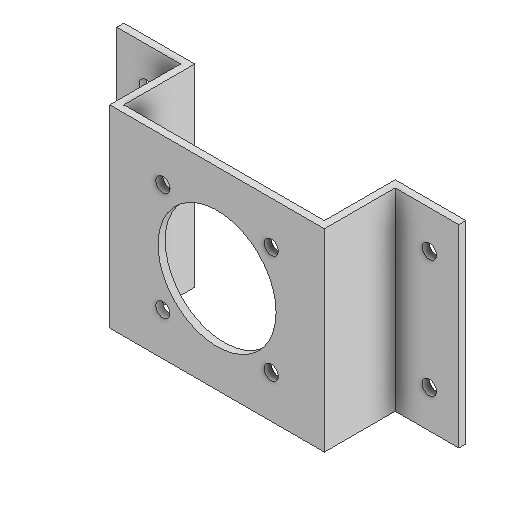
# Autodesk Inventor part: TopMotorBracket
Saved by Autodesk Inventor 2022 (Build 260153000, 153)
## iProperties
Created: 2024-07-02
Part Number: TopMotorBracket
Material: Generic
Document SubType Name: Modeling
Designer: LaptopJR
Density: 1 g/cm^3
Appearance: Default
Author: LaptopJR
Autodesk Inventor part; units mm, degrees
ref_plane "YZ Plane" through (0, 0, 0) normal (1, 0, 0) x (0, 1, 0)
ref_plane "XZ Plane" through (0, 0, 0) normal (0, 1, 0) x (-1, 0, 0)
ref_plane "XY Plane" through (0, 0, 0) normal (0, 0, 1) x (1, 0, 0)
sketch "Sketch1" plane through (0, 0, 0) normal (0, 1, 0) x (-1, 0, 0)
  line L0 (0, 0) -> (-30, 0)
  line L1 (-30, 0) -> (-30, 30)
  line L2 (-30, 30) -> (-115, 30)
  line L3 (-115, 30) -> (-115, 0)
  line L4 (-115, 0) -> (-145, 0)
  line L5 (0, 3) -> (-27, 3)
  line L6 (-27, 3) -> (-27, 33)
  line L7 (-27, 33) -> (-118, 33)
  line L8 (-118, 33) -> (-118, 3)
  line L9 (-118, 3) -> (-145, 3)
  line L10 (0, 0) -> (0, 3)
  line L11 (-145, 0) -> (-145, 3)
  dimension "d0" = 30
  dimension "d1" = 30
  dimension "d2" = 3
  dimension "d28" = 85
  constraints: 24 end point, 6 perpendicular, 2 point on line, 2 vertical, 1 collinear, 1 horizontal, 4 other
  measures "d0" distance of L0.start L0.end
  measures "d1" distance of L0.end L1.end
  measures "d2" distance between parallel lines of L2 L7
  measures "d28" distance of L1.end L2.end
extrude "Extrusion1" add sketch "Sketch1" along normal blind 82
sketch "Sketch2" plane through (27, 0, 33) normal (0, 0, 1) x (1, 0, 0)
  line L0 (0, 82) -> (91, 82) projected
  line L1 (45.5, 82) -> (45.5, 0) construction
  line L2 (0, 0) -> (91, 0) projected
  circle A0 centre (45.5, 41) radius 32.5 construction
  line L3 (45.5, 41) -> (68.481, 63.981) construction
  circle A1 centre (68.481, 63.981) radius 3.05
  circle A2 centre (22.519, 63.981) radius 3.05
  circle A3 centre (22.519, 18.019) radius 3.05
  circle A4 centre (68.481, 18.019) radius 3.05
  circle A5 centre (45.5, 41) radius 25.0125
  point P0 (-27, 0)
  dimension "d6" = 65
  dimension "d7" = 6.1
  dimension "d8" = 45
  dimension "d11" = 360
  dimension "d15" = 50.025
  constraints: 5 centre point, 4 end point, 3 midpoint, 2 coincident, 12 other
  measures "d7" diameter of A1
  measures "d8" angle of L1 L3
  measures "d15" diameter of A5
extrude "Extrusion2" cut sketch "Sketch2" against normal blind 82
sketch "Sketch3" plane through (0, 0, 3) normal (0, 0, 1) x (1, 0, 0)
  circle A0 centre (72.5, 41) radius 25.0125 construction
  line L0 (12.5, 66) -> (132.5, 66) construction
  line L1 (132.5, 66) -> (132.5, 16) construction
  line L2 (132.5, 16) -> (12.5, 16) construction
  line L3 (12.5, 16) -> (12.5, 66) construction
  line L4 (12.5, 66) -> (132.5, 16) construction
  line L5 (132.5, 66) -> (12.5, 16) construction
  circle A1 centre (12.5, 66) radius 3.05
  circle A2 centre (12.5, 16) radius 3.05
  circle A3 centre (132.5, 66) radius 3.05
  circle A4 centre (132.5, 16) radius 3.05
  dimension "d29" = 6.1
  dimension "d30" = 120
  dimension "d31" = 50
  constraints: 12 end point, 4 centre point, 4 coincident, 3 equal radius, 2 midpoint, 2 parallel, 1 horizontal, 1 perpendicular
  measures "d29" diameter of A1
  measures "d30" distance of L0.start L0.end
  measures "d31" distance of L2.end L0.start
extrude "Extrusion3" cut sketch "Sketch3" against normal blind 10
body "Solid1"
